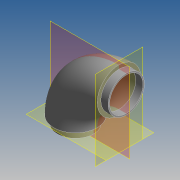
# Autodesk Inventor part: P010_CanonCoude
Saved by Autodesk Inventor 2020 (Build 240168000, 168)
## iProperties
Created: 2021-10-15
Part Number: P010_CanonCoude
Material: Générique
Document SubType Name: Modeling
Designer: gabri
Density: 1 g/cm^3
Appearance: Par défaut
Author: gabri
Autodesk Inventor part; units mm, degrees
sketch "Esquisse15" plane through (0, 0, 0) normal (1, 0, 0) x (0, 1, 0)
  circle A0 centre (0, 60) radius 30
  circle A1 centre (0, 60) radius 23
  line L0 (-42, 0) -> (42, 0) construction
  line L1 (0, 108) -> (0, -18) construction
  point P0 (0, 0)
  dimension "d43" = 60
  dimension "d44" = 46
  dimension "d45" = 60
  constraints: 2 centre point, 1 coincident, 1 point on line
  measures "d43" diameter of A0
  measures "d44" diameter of A1
  measures "d45" distance from line of L0 A0.centre
sketch "Esquisse9" plane through (0, 0, 0) normal (0, 1, 0) x (-1, 0, 0)
  arc A0 (60, 0) -> (0, 60) centre (0, 0) ccw
  dimension "d41" = 90
  dimension "d42" = 60
  constraints: 2 point on circle, 1 centre point, 1 coincident
  measures "d42" distance of point (0, 0) A0.start
sweep "Balayage3" add profiles "Esquisse15" path "Esquisse9"
sketch "Esquisse16" plane through (-60, 0, 0) normal (0, 0, -1) x (-1, 0, 0)
  circle A0 centre (0, 0) radius 23 construction
  circle A1 centre (0, 0) radius 30 construction
  circle A2 centre (0, 0) radius 23
  circle A3 centre (0, 0) radius 25
  point P0 (-60, 0)
  dimension "d48" = 50
  constraints: 2 centre point, 2 coincident, 1 concentric
  measures "d48" diameter of A3
extrude "Extrusion6" add sketch "Esquisse16" along normal blind 10
sketch "Esquisse17" plane through (0, 0, 60) normal (1, 0, 0) x (0, 0, -1)
  circle A0 centre (0, 0) radius 23 construction
  circle A1 centre (0, 0) radius 30 construction
  circle A2 centre (0, 0) radius 23
  circle A3 centre (0, 0) radius 25
  point P0 (60, 0)
  dimension "d51" = 50
  constraints: 2 centre point, 2 coincident, 1 concentric
  measures "d51" diameter of A3
extrude "Extrusion7" add sketch "Esquisse17" along normal blind 10
